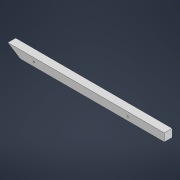
# Autodesk Inventor part: freio rolimã, como tu e tua irmã
Saved by Autodesk Inventor 2022 (Build 260153000, 153)
## iProperties
Created: 2022-06-10
Part Number: freio rolimã, como tu e tua irmã
Material: Genérico
Document SubType Name: Modeling
Designer: jonat
Density: 1 g/cm^3
Appearance: Padrão
Author: jonat
Autodesk Inventor part; units mm, degrees
ref_plane "YZ Plane" through (0, 0, 0) normal (1, 0, 0) x (0, 1, 0)
ref_plane "XZ Plane" through (0, 0, 0) normal (0, 1, 0) x (-1, 0, 0)
ref_plane "XY Plane" through (0, 0, 0) normal (0, 0, 1) x (1, 0, 0)
sketch "Esboço1" plane through (0, 0, 0) normal (1, 0, 0) x (0, 1, 0)
  line L0 (3.7958, 6.2827) -> (-21.2042, 6.2827)
  line L1 (-21.2042, 6.2827) -> (-21.2042, -18.7173)
  line L2 (-21.2042, -18.7173) -> (3.7958, -18.7173)
  line L3 (3.7958, -18.7173) -> (3.7958, 6.2827)
  point P0 (0, 0)
  dimension "d0" = 25
  dimension "d1" = 25
  constraints: 8 end point, 2 parallel, 1 horizontal, 1 perpendicular
  measures "d0" distance of L2.end L1.end
  measures "d1" distance of L1.end L0.end
extrude "Extrusão1" add sketch "Esboço1" along normal blind 500
sketch "Esboço2" plane through (0, -21.2042, 6.2827) normal (0, 0, 1) x (1, 0, 0)
  line L0 (0, 25) -> (500, 25) projected
  line L1 (0, 0) -> (0, 25) projected
  line L2 (0, 25) -> (0, 0)
  line L3 (0, 0) -> (39.6735, 0)
  line L4 (0, 0) -> (500, 0) projected
  line L5 (0, 25) -> (39.6735, 0)
  point P0 (0, 21.2042)
  constraints: 6 end point, 1 collinear, 1 point on line
extrude "Extrusão2" cut sketch "Esboço2" against normal blind 25
sketch "Esboço3" plane through (500, -21.2042, -18.7173) normal (0, 0, -1) x (-1, 0, 0)
  circle A0 centre (116.1656, 12.3184) radius 2.5
  point P0 (500, 21.2042)
  dimension "d6" = 5
  constraints: 1 centre point
  measures "d6" diameter of A0
extrude "Extrusão3" cut sketch "Esboço3" against normal blind 25
sketch "Sketch4" plane through (500, -21.2042, 6.2827) normal (0, 0, 1) x (1, 0, 0)
  circle A0 centre (-416.7971, 13.0246) radius 2.5
  point P0 (-500, 21.2042)
  dimension "d9" = 5
  constraints: 1 centre point
  measures "d9" diameter of A0
extrude "Extrusion4" cut sketch "Sketch4" against normal blind 25
